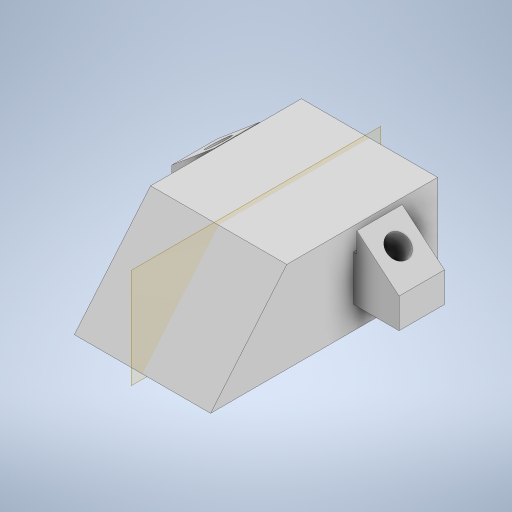
# Autodesk Inventor part: taslak
Saved by Autodesk Inventor 2023 (Build 270158000, 158)
## iProperties
Created: 2023-03-22
Part Number: taslak
Material: Generic
Document SubType Name: Modeling
Designer: Umut Yücesoy
Density: 1 g/cm^3
Appearance: Default
Author: Umut Yücesoy
Autodesk Inventor part; units mm, degrees
ref_plane "YZ Plane" through (0, 0, 0) normal (1, 0, 0) x (0, 1, 0)
ref_plane "XZ Plane" through (0, 0, 0) normal (0, 1, 0) x (-1, 0, 0)
ref_plane "XY Plane" through (0, 0, 0) normal (0, 0, 1) x (1, 0, 0)
sketch "Sketch1" plane through (0, 0, 0) normal (0, 1, 0) x (-1, 0, 0)
  line L0 (0, 0) -> (60, 0)
  line L1 (60, 0) -> (60, -100)
  line L2 (60, -100) -> (0, -100)
  line L3 (0, -100) -> (0, 0)
  dimension "d0" = 100
  dimension "d1" = 60
  constraints: 8 end point, 2 parallel, 1 horizontal, 1 perpendicular
  measures "d0" distance of L0.end L1.end
  measures "d1" distance of L1.end L2.end
extrude "Extrusion1" add sketch "Sketch1" along normal blind 40
sketch "Sketch2" plane through (0, 0, 0) normal (1, 0, 0) x (0, 0, -1)
  line L0 (0, 0) -> (37.6485, 44.8677)
  line L1 (0, 0) -> (58.5706, 0) construction
  line L2 (100, 40) -> (0, 40) projected
  line L3 (0, 40) -> (0, 0)
  point P0 (33.564, 40)
  dimension "d4" = 50
  constraints: 6 end point, 1 equal length, 1 horizontal, 1 perpendicular
  measures "d4" angle of L1 L0
extrude "Extrusion2" cut sketch "Sketch2" against normal blind 70
sketch "Sketch3" plane through (0, 0, -100) normal (1, 0, 0) x (0, 0, -1)
  line L0 (0, 0) -> (-17, 0)
  line L1 (-100, 0) -> (0, 0) projected
  line L2 (0, 40) -> (-66.436, 40) projected
  line L3 (-17, 40) -> (-37, 40)
  line L4 (-37, 40) -> (-37, 10)
  line L5 (-37, 10) -> (-17, 10)
  line L6 (-17, 10) -> (-17, 40)
  dimension "d7" = 17
  dimension "d8" = 20
  dimension "d9" = 30
  constraints: 10 end point, 3 point on line, 1 parallel, 1 perpendicular, 1 vertical
  measures "d7" distance of L0.start L0.end
  measures "d8" distance of L3.start L3.end
  measures "d9" distance of L3.end L4.end
extrude "Extrusion3" add sketch "Sketch3" along normal blind 20
sketch "Sketch4" plane through (0, 10, -63) normal (0, 0, 1) x (1, 0, 0)
  line L0 (0, 30) -> (-60, 30) projected
  line L1 (0, 30) -> (29.4147, 5.3181)
  line L2 (0, 30) -> (38.3982, 30) construction
  line L3 (0, 30) -> (20, 30) projected
  line L4 (0, 30) -> (20, 30)
  line L5 (20, 30) -> (20, 13.218)
  line L6 (20, 0) -> (20, 30) projected
  point P0 (0, -10)
  dimension "d12" = 40
  constraints: 8 end point, 4 point on line, 1 collinear, 1 equal length, 1 horizontal
  measures "d12" angle of L1 L2
extrude "Extrusion4" cut sketch "Sketch4" against normal blind 61.75
ref_plane "Work Plane1" through (-30, 0, -100) normal (1, 0, 0) x (0, 0, -1)
mirror "Mirror1" about plane through (-30, 0, -100) normal (1, 0, 0) of "Extrusion3", "Extrusion4"
sketch "Sketch5" plane through (0, 40, -63) normal (0.6428, 0.766, 0) x (0.766, -0.6428, 0)
  circle A0 centre (12.5, 10) radius 5
  point P0 (25.7115, -63)
  dimension "d16" = 10
  constraints: 1 centre point
  measures "d16" diameter of A0
extrude "Extrusion5" cut sketch "Sketch5" against normal blind 27
mirror "Mirror2" about plane through (-30, 0, -100) normal (1, 0, 0) of "Extrusion5"
sketch "Sketch6" plane through (20, 10, -83) normal (0, 0, -1) x (-1, 0, 0)
  line L0 (20, 30) -> (20, 0) projected
  line L1 (20, 30) -> (20, 20)
  line L2 (20, 20) -> (18.6004, 20)
  line L3 (18.6004, 20) -> (18.6004, 28.8256)
  line L4 (0, 13.218) -> (20, 30) projected
  point P0 (20, -10)
  point P1 (20, 20)
  dimension "d19" = 10
  constraints: 6 end point, 2 perpendicular, 1 point on line, 1 vertical
  measures "d19" distance of L0.start L1.end
extrude "Extrusion6" cut sketch "Sketch6" against normal blind 38.25
mirror "Mirror3" about plane through (-30, 0, -100) normal (1, 0, 0) of "Extrusion6"
body "Solid1"
